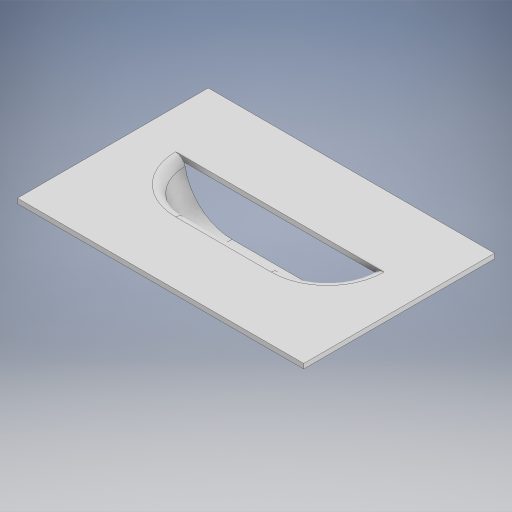
# Autodesk Inventor part: CE-4.1.2
Saved by Autodesk Inventor 2024 (Build 280153000, 153)
## iProperties
Created: 2024-02-08
Part Number: CE-4.1.2
Material: Generic
Document SubType Name: Sheet Metal
Designer: Alex
Density: 1 g/cm^3
Sheet Metal Rule: Default_mm
Appearance: Default
Author: Alex
Autodesk Inventor part; units mm, degrees
ref_plane "YZ Plane" through (0, 0, 0) normal (1, 0, 0) x (0, 1, 0)
ref_plane "XZ Plane" through (0, 0, 0) normal (0, 1, 0) x (-1, 0, 0)
sketch "Sketch1" plane through (0, 0, 0) normal (0, 1, 0) x (-1, 0, 0)
  line L0 (0, 0) -> (-30, 0)
  line L1 (-30, 0) -> (-30, -20)
  line L2 (-30, -20) -> (0, -20)
  line L3 (0, -20) -> (0, 0)
  dimension "d0" = 30
  dimension "d1" = 20
  measures "d0" distance of L1.end L2.end
  measures "d1" distance of L0.end L1.end
extrude "Plate1" add sketch "Sketch1" along normal blind 0.5
sketch "Sketch2" plane through (0, 0.5, 0) normal (0, 1, 0) x (1, 0, 0)
  arc A0 (5, 12.5) -> (10, 7.5) centre (10, 12.5) ccw
  line L0 (10, 7.5) -> (20, 7.5)
  arc A1 (20, 7.5) -> (25, 12.5) centre (20, 12.5) ccw
  line L1 (5, 12.5) -> (25, 12.5)
  line L2 (15, 12.5) -> (15, 7.5) construction
  line L3 (30, 0) -> (0, 0) construction
  line L4 (0, 0) -> (0, 20) construction
  point P0 (15, 10)
  dimension "d3" = 20
  dimension "d4" = 5
  dimension "d5" = 10
  dimension "d6" = 15
  constraints: 6 end point, 4 point on circle, 3 midpoint, 2 centre point, 2 horizontal, 2 point on line, 1 equal radius, 1 tangent
  measures "d3" distance of L1.start L1.end
  measures "d4" radius of A0
  measures "d5" distance from line of L3 point (15, 10)
  measures "d6" distance from line of L4 point (15, 10)
extrude "Extrusion1" cut sketch "Sketch2" against normal blind 0.5
ref_plane "Work Plane1" through (10, 0.5, -12.5) normal (0, -1, 0) x (1, 0, 0)
sketch "Sketch3" plane through (10, 0.5, -12.5) normal (0, -1, 0) x (1, 0, 0)
  arc A0 (0, 5) -> (-5, 0) centre (0, 0) ccw projected
  line L0 (-5, 0) -> (15, 0) projected
  line L1 (10, 5) -> (0, 5) projected
  arc A1 (15, 0) -> (10, 5) centre (10, 0) ccw projected
  line L2 (5, 0) -> (5, 5) construction
  line L3 (15, 0) -> (-5, 0) projected
  line L4 (-5, 0) -> (-5.5, 0)
  arc A2 (0, 5.5) -> (-5.5, 0) centre (0, 0) ccw
  line L5 (0, 5.5) -> (10, 5.5)
  arc A3 (15.5, 0) -> (10, 5.5) centre (10, 0) ccw
  line L6 (15.5, 0) -> (15, 0)
  point P0 (-10, 12.5)
  dimension "d9" = 0.5
  constraints: 6 end point, 4 point on circle, 2 centre point, 2 concentric, 2 horizontal, 2 tangent, 1 point on line
  measures "d9" distance of L0.start L4.end
revolve "Revolution1" add sketch "Sketch3" angle 90 about axis through (5, 0.5, -12.5) along (1, 0, 0) contours A0 L4 A2 L5 A3 L6 A1 L1
fillet "Fillet1" radius 1 6 edges at (6.4645, 0.5, -8.9645) (23.5355, 0.5, -8.9645) (15, 0.5, -7.5) (23.873, 0, -8.627) (6.127, 0, -8.627) (15, 0, -7.0228)
equation "\"d7\" = Thickness"
equation "\"d9\" = Thickness"
equation "\"d2\" = Thickness"
equation "\"BendRadius\" = Thickness"
equation "\"BendReliefWidth\" = Thickness"
equation "\"BendReliefDepth\" = 0.5 * Thickness"
equation "\"CornerReliefSize\" = 4 * Thickness"
equation "\"MinimumRemnant\" = 2 * Thickness"
equation "\"TransitionRadius\" = BendRadius"
equation "\"JacobiRadiusSize\" = BendRadius"
equation "\"GapSize\" = Thickness"
equation "\"Thickness\" = 0.5"
body "Solid1"
